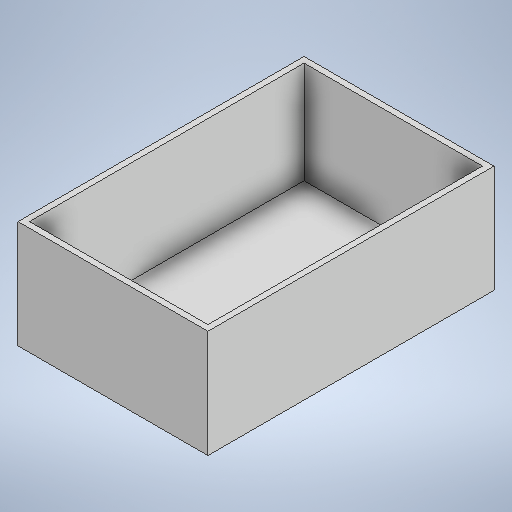
# Autodesk Inventor part: box_under
Saved by Autodesk Inventor 2025.2 (Build 292293000, 293)
## iProperties
Created: 2025-02-21
Part Number: box_under
Material: Generic
Document SubType Name: Modeling
Designer: fiste
Density: 1 g/cm^3
Appearance: Default
Author: fiste
Autodesk Inventor part; units mm, degrees
ref_plane "YZ Plane" through (0, 0, 0) normal (1, 0, 0) x (0, 1, 0)
ref_plane "XZ Plane" through (0, 0, 0) normal (0, 1, 0) x (-1, 0, 0)
ref_plane "XY Plane" through (0, 0, 0) normal (0, 0, 1) x (1, 0, 0)
sketch "Sketch1" plane through (0, 0, 0) normal (0, 0, 1) x (1, 0, 0)
  line L0 (0, 0) -> (330, 0)
  line L1 (330, 0) -> (330, 497)
  line L2 (330, 497) -> (0, 497)
  line L3 (0, 497) -> (0, 0)
  dimension "d0" = 330
  dimension "d1" = 497
  constraints: 8 end point, 2 parallel, 1 horizontal, 1 perpendicular
  measures "d0" distance of L2.end L1.end
  measures "d1" distance of L1.end L0.end
extrude "Extrusion1" add sketch "Sketch1" along normal blind 10
sketch "Sketch2" plane through (0, 0, 10) normal (0, 0, 1) x (1, 0, 0)
  line L0 (0, 0) -> (330, 0)
  line L1 (330, 0) -> (330, 497)
  line L2 (330, 497) -> (0, 497)
  line L3 (0, 497) -> (0, 0)
  line L4 (10, 487) -> (320, 487)
  line L5 (320, 487) -> (320, 10)
  line L6 (320, 10) -> (10, 10)
  line L7 (10, 10) -> (10, 487)
  dimension "d4" = 330
  dimension "d5" = 497
  dimension "d6" = 10
  constraints: 16 end point, 4 parallel, 2 perpendicular, 1 horizontal, 3 other
  measures "d4" distance of L2.end L1.end
  measures "d5" distance of L1.end L0.end
  measures "d6" distance between parallel lines of L2 L4
extrude "Extrusion2" add sketch "Sketch2" along normal blind 177
body "Solid1"
